Autodesk Fusion 360 part; units mm, degrees
(part 7 of 8)
  spline S2095 degree 3 poles (9.9865, -104.511) (10.0552, -104.4975) (10.0546, -104.4926) (9.9819, -104.494) knots 0 0 0 0 1 1 1 1
  spline S2096 degree 3 poles (9.9819, -104.494) (9.9092, -104.4954) (9.8779, -104.5067) (9.9001, -104.5241) knots 0 0 0 0 1 1 1 1
  spline S2097 degree 3 poles (10.4842, -104) (10.5266, -103.9973) (10.5607, -103.9881) (10.5588, -103.9733) knots 0 0 0 0 1 1 1 1
  spline S2098 degree 3 poles (10.5588, -103.9733) (10.557, -103.9584) (10.5998, -103.9381) (10.6487, -103.927) knots 0 0 0 0 1 1 1 1
  spline S2099 degree 3 poles (10.6487, -103.927) (10.7443, -103.9078) (10.7443, -103.9078) (10.6391, -103.9106) knots 0 0 0 0 1 1 1 1
  spline S2100 degree 3 poles (10.6391, -103.9106) (10.5819, -103.9151) (10.5379, -103.9256) (10.5397, -103.9404) knots 0 0 0 0 1 1 1 1
  spline S2101 degree 3 poles (10.5397, -103.9404) (10.5415, -103.9553) (10.5109, -103.9716) (10.4719, -103.9814) knots 0 0 0 0 1 1 1 1
  spline S2102 degree 3 poles (10.4719, -103.9814) (10.4109, -103.9964) (10.4137, -103.9986) (10.4842, -104) knots 0 0 0 0 1 1 1 1
  spline S2103 degree 3 poles (11.4822, -102.6711) (11.4877, -102.6755) (11.5273, -102.6706) (11.5685, -102.658) knots 0 0 0 0 1 1 1 1
  spline S2104 degree 3 poles (11.5685, -102.658) (11.6372, -102.6445) (11.6366, -102.6396) (11.5639, -102.641) knots 0 0 0 0 1 1 1 1
  spline S2105 degree 3 poles (11.5639, -102.641) (11.4912, -102.6424) (11.4599, -102.6537) (11.4822, -102.6711) knots 0 0 0 0 1 1 1 1
  spline S2106 degree 3 poles (12.3845, -101.6078) (12.4368, -101.6039) (12.4836, -101.5956) (12.4879, -101.5901) knots 0 0 0 0 1 1 1 1
  spline S2107 degree 3 poles (12.4879, -101.5901) (12.4923, -101.5845) (12.4586, -101.5761) (12.4128, -101.5717) knots 0 0 0 0 1 1 1 1
  spline S2108 degree 3 poles (12.4128, -101.5717) (12.367, -101.5672) (12.3203, -101.5755) (12.3094, -101.5894) knots 0 0 0 0 1 1 1 1
  spline S2109 degree 3 poles (12.3094, -101.5894) (12.2985, -101.6033) (12.3322, -101.6117) (12.3845, -101.6078) knots 0 0 0 0 1 1 1 1
  spline S2110 degree 3 poles (8.4693, -106.5847) (8.4748, -106.5891) (8.5145, -106.5842) (8.5556, -106.5716) knots 0 0 0 0 1 1 1 1
  spline S2111 degree 3 poles (8.5556, -106.5716) (8.6243, -106.5582) (8.6237, -106.5532) (8.551, -106.5546) knots 0 0 0 0 1 1 1 1
  spline S2112 degree 3 poles (8.551, -106.5546) (8.4783, -106.556) (8.447, -106.5674) (8.4693, -106.5847) knots 0 0 0 0 1 1 1 1
  spline S2113 degree 3 poles (15.3364, -97.8927) (15.3503, -97.9035) (15.3667, -97.894) (15.3692, -97.8736) knots 0 0 0 0 1 1 1 1
  spline S2114 degree 3 poles (15.3692, -97.8736) (15.3739, -97.8504) (15.3687, -97.8284) (15.3603, -97.8219) knots 0 0 0 0 1 1 1 1
  spline S2115 degree 3 poles (15.3603, -97.8219) (15.3548, -97.8175) (15.3405, -97.8243) (15.3275, -97.841) knots 0 0 0 0 1 1 1 1
  spline S2116 degree 3 poles (15.3275, -97.841) (15.3166, -97.8549) (15.3197, -97.8797) (15.3364, -97.8927) knots 0 0 0 0 1 1 1 1
  spline S2117 degree 3 poles (11.7356, -102.6677) (11.7879, -102.6637) (11.8346, -102.6555) (11.8411, -102.6472) knots 0 0 0 0 1 1 1 1
  spline S2118 degree 3 poles (11.8411, -102.6472) (11.8476, -102.6388) (11.8096, -102.6359) (11.7573, -102.6399) knots 0 0 0 0 1 1 1 1
  spline S2119 degree 3 poles (11.7573, -102.6399) (11.705, -102.6438) (11.6583, -102.652) (11.6517, -102.6604) knots 0 0 0 0 1 1 1 1
  spline S2120 degree 3 poles (11.6517, -102.6604) (11.6452, -102.6687) (11.6833, -102.6716) (11.7356, -102.6677) knots 0 0 0 0 1 1 1 1
  spline S2121 degree 3 poles (10.6627, -104.0007) (10.6683, -104.0051) (10.7036, -104.0058) (10.7376, -103.9965) knots 0 0 0 0 1 1 1 1
  spline S2122 degree 3 poles (10.7376, -103.9965) (10.7865, -103.9855) (10.7974, -103.9716) (10.7826, -103.9332) knots 0 0 0 0 1 1 1 1
  spline S2123 degree 3 poles (10.7826, -103.9332) (10.7718, -103.9069) (10.7635, -103.9004) (10.7638, -103.923) knots 0 0 0 0 1 1 1 1
  spline S2124 degree 3 poles (10.7638, -103.923) (10.7662, -103.9428) (10.7417, -103.9684) (10.7076, -103.9776) knots 0 0 0 0 1 1 1 1
  spline S2125 degree 3 poles (10.7076, -103.9776) (10.6758, -103.984) (10.6544, -103.9942) (10.6627, -104.0007) knots 0 0 0 0 1 1 1 1
  spline S2126 degree 3 poles (11.3676, -103.2532) (11.3815, -103.264) (11.4063, -103.261) (11.4172, -103.2471) knots 0 0 0 0 1 1 1 1
  spline S2127 degree 3 poles (11.4172, -103.2471) (11.4302, -103.2304) (11.425, -103.2084) (11.4111, -103.1976) knots 0 0 0 0 1 1 1 1
  spline S2128 degree 3 poles (11.4111, -103.1976) (11.3944, -103.1845) (11.3746, -103.187) (11.3616, -103.2037) knots 0 0 0 0 1 1 1 1
  spline S2129 degree 3 poles (11.3616, -103.2037) (11.3507, -103.2176) (11.351, -103.2401) (11.3676, -103.2532) knots 0 0 0 0 1 1 1 1
  spline S2130 degree 3 poles (12.6924, -101.5976) (12.741, -101.6042) (12.7806, -101.5994) (12.7788, -101.5845) knots 0 0 0 0 1 1 1 1
  spline S2131 degree 3 poles (12.7788, -101.5845) (12.7797, -101.5718) (12.7389, -101.5668) (12.6894, -101.5729) knots 0 0 0 0 1 1 1 1
  spline S2132 degree 3 poles (12.6894, -101.5729) (12.608, -101.5854) (12.6058, -101.5882) (12.6924, -101.5976) knots 0 0 0 0 1 1 1 1
  spline S2133 degree 3 poles (14.4902, -99.2909) (14.5124, -99.3083) (14.5344, -99.3031) (14.5369, -99.2827) knots 0 0 0 0 1 1 1 1
  spline S2134 degree 3 poles (14.5369, -99.2827) (14.5388, -99.2573) (14.5237, -99.2365) (14.5033, -99.234) knots 0 0 0 0 1 1 1 1
  spline S2135 degree 3 poles (14.5033, -99.234) (14.4448, -99.2286) (14.4401, -99.2518) (14.4902, -99.2909) knots 0 0 0 0 1 1 1 1
  spline S2136 degree 3 poles (10.9505, -103.8674) (10.956, -103.8717) (10.9956, -103.8668) (11.0368, -103.8542) knots 0 0 0 0 1 1 1 1
  spline S2137 degree 3 poles (11.0368, -103.8542) (11.1055, -103.8408) (11.1049, -103.8358) (11.0322, -103.8372) knots 0 0 0 0 1 1 1 1
  spline S2138 degree 3 poles (11.0322, -103.8372) (10.9595, -103.8386) (10.9282, -103.85) (10.9505, -103.8674) knots 0 0 0 0 1 1 1 1
  spline S2139 degree 3 poles (11.9636, -102.6623) (12.1053, -102.67) (12.929, -102.6644) (12.9983, -102.6559) knots 0 0 0 0 1 1 1 1
  spline S2140 degree 3 poles (12.9983, -102.6559) (13.1066, -102.6375) (13.0389, -102.6383) (12.4983, -102.6368) knots 0 0 0 0 1 1 1 1
  spline S2141 degree 3 poles (12.4983, -102.6368) (12.0911, -102.6366) (11.7888, -102.6511) (11.9636, -102.6623) knots 0 0 0 0 1 1 1 1
  spline S2142 degree 3 poles (8.921, -106.5795) (8.9266, -106.5839) (8.9662, -106.579) (9.0074, -106.5664) knots 0 0 0 0 1 1 1 1
  spline S2143 degree 3 poles (9.0074, -106.5664) (9.0761, -106.553) (9.0755, -106.548) (9.0028, -106.5494) knots 0 0 0 0 1 1 1 1
  spline S2144 degree 3 poles (9.0028, -106.5494) (8.9301, -106.5508) (8.8988, -106.5622) (8.921, -106.5795) knots 0 0 0 0 1 1 1 1
  spline S2145 degree 3 poles (10.9843, -103.9386) (10.9899, -103.9429) (11.0295, -103.9381) (11.0707, -103.9255) knots 0 0 0 0 1 1 1 1
  spline S2146 degree 3 poles (11.0707, -103.9255) (11.1394, -103.912) (11.1388, -103.9071) (11.0661, -103.9085) knots 0 0 0 0 1 1 1 1
  spline S2147 degree 3 poles (11.0661, -103.9085) (10.9934, -103.9098) (10.9621, -103.9212) (10.9843, -103.9386) knots 0 0 0 0 1 1 1 1
  spline S2148 degree 3 poles (11.5768, -103.2375) (11.5824, -103.2419) (11.622, -103.237) (11.6632, -103.2244) knots 0 0 0 0 1 1 1 1
  spline S2149 degree 3 poles (11.6632, -103.2244) (11.7319, -103.211) (11.7313, -103.206) (11.6586, -103.2074) knots 0 0 0 0 1 1 1 1
  spline S2150 degree 3 poles (11.6586, -103.2074) (11.5859, -103.2088) (11.5546, -103.2202) (11.5768, -103.2375) knots 0 0 0 0 1 1 1 1
  spline S2151 degree 3 poles (11.1371, -103.9952) (11.1541, -103.9906) (11.1869, -103.9715) (11.2071, -103.9515) knots 0 0 0 0 1 1 1 1
  spline S2152 degree 3 poles (11.2071, -103.9515) (11.2294, -103.9286) (11.2353, -103.9153) (11.2177, -103.915) knots 0 0 0 0 1 1 1 1
  spline S2153 degree 3 poles (11.2177, -103.915) (11.2007, -103.9196) (11.1678, -103.9387) (11.1477, -103.9588) knots 0 0 0 0 1 1 1 1
  spline S2154 degree 3 poles (11.1477, -103.9588) (11.1253, -103.9816) (11.1194, -103.9949) (11.1371, -103.9952) knots 0 0 0 0 1 1 1 1
  spline S2155 degree 3 poles (11.9296, -103.2445) (11.9351, -103.2488) (11.9747, -103.244) (12.0159, -103.2314) knots 0 0 0 0 1 1 1 1
  spline S2156 degree 3 poles (12.0159, -103.2314) (12.0846, -103.2179) (12.084, -103.213) (12.0113, -103.2144) knots 0 0 0 0 1 1 1 1
  spline S2157 degree 3 poles (12.0113, -103.2144) (11.9386, -103.2157) (11.9073, -103.2271) (11.9296, -103.2445) knots 0 0 0 0 1 1 1 1
  line L166 (17.1117, -96.7951) -> (17.1249, -96.9845)
  line L167 (17.1249, -96.9845) -> (17.1293, -96.7954)
  spline S2158 degree 3 poles (17.1293, -96.7954) (17.1324, -96.6367) (17.1245, -96.5723) (17.105, -96.5973) knots 0 0 0 0 1 1 1 1
  spline S2159 degree 3 poles (17.105, -96.5973) (17.1006, -96.6029) (17.1038, -96.6905) (17.1117, -96.7951) knots 0 0 0 0 1 1 1 1
  spline S2160 degree 3 poles (11.5786, -103.8656) (11.5841, -103.87) (11.6237, -103.8651) (11.6649, -103.8525) knots 0 0 0 0 1 1 1 1
  spline S2161 degree 3 poles (11.6649, -103.8525) (11.7336, -103.8391) (11.733, -103.8341) (11.6603, -103.8355) knots 0 0 0 0 1 1 1 1
  spline S2162 degree 3 poles (11.6603, -103.8355) (11.5876, -103.8369) (11.5563, -103.8483) (11.5786, -103.8656) knots 0 0 0 0 1 1 1 1
  spline S2163 degree 3 poles (13.3873, -101.6078) (13.3929, -101.6122) (13.4325, -101.6073) (13.4737, -101.5947) knots 0 0 0 0 1 1 1 1
  spline S2164 degree 3 poles (13.4737, -101.5947) (13.5424, -101.5812) (13.5418, -101.5763) (13.4691, -101.5777) knots 0 0 0 0 1 1 1 1
  spline S2165 degree 3 poles (13.4691, -101.5777) (13.3964, -101.5791) (13.3651, -101.5904) (13.3873, -101.6078) knots 0 0 0 0 1 1 1 1
  spline S2166 degree 3 poles (12.1554, -103.2419) (12.161, -103.2462) (12.2006, -103.2414) (12.2418, -103.2288) knots 0 0 0 0 1 1 1 1
  spline S2167 degree 3 poles (12.2418, -103.2288) (12.3105, -103.2153) (12.3099, -103.2104) (12.2372, -103.2118) knots 0 0 0 0 1 1 1 1
  spline S2168 degree 3 poles (12.2372, -103.2118) (12.1645, -103.2131) (12.1332, -103.2245) (12.1554, -103.2419) knots 0 0 0 0 1 1 1 1
  spline S2169 degree 3 poles (7.6066, -109.1788) (7.6121, -109.1831) (7.6517, -109.1783) (7.6929, -109.1657) knots 0 0 0 0 1 1 1 1
  spline S2170 degree 3 poles (7.6929, -109.1657) (7.7616, -109.1522) (7.761, -109.1473) (7.6883, -109.1486) knots 0 0 0 0 1 1 1 1
  spline S2171 degree 3 poles (7.6883, -109.1486) (7.6156, -109.15) (7.5843, -109.1614) (7.6066, -109.1788) knots 0 0 0 0 1 1 1 1
  spline S2172 degree 3 poles (11.832, -103.8622) (11.8843, -103.8583) (11.931, -103.85) (11.9375, -103.8417) knots 0 0 0 0 1 1 1 1
  spline S2173 degree 3 poles (11.9375, -103.8417) (11.944, -103.8333) (11.906, -103.8305) (11.8537, -103.8344) knots 0 0 0 0 1 1 1 1
  spline S2174 degree 3 poles (11.8537, -103.8344) (11.8014, -103.8383) (11.7547, -103.8465) (11.7481, -103.8549) knots 0 0 0 0 1 1 1 1
  spline S2175 degree 3 poles (11.7481, -103.8549) (11.7416, -103.8632) (11.7797, -103.8661) (11.832, -103.8622) knots 0 0 0 0 1 1 1 1
  line L168 (17.1131, -97.1141) -> (17.1358, -97.2168)
  line L169 (17.1358, -97.2168) -> (17.1329, -97.1116)
  spline S2176 degree 3 poles (17.1329, -97.1116) (17.1284, -97.0544) (17.1223, -97.0049) (17.1168, -97.0005) knots 0 0 0 0 1 1 1 1
  spline S2177 degree 3 poles (17.1168, -97.0005) (17.0945, -96.9832) (17.0938, -97.0184) (17.1131, -97.1141) knots 0 0 0 0 1 1 1 1
  spline S2178 degree 3 poles (13.3509, -101.9868) (13.4258, -101.9826) (13.4983, -101.9586) (13.5129, -101.9342) knots 0 0 0 0 1 1 1 1
  spline S2179 degree 3 poles (13.5129, -101.9342) (13.5433, -101.8953) (13.5405, -101.8931) (13.4984, -101.9184) knots 0 0 0 0 1 1 1 1
  spline S2180 degree 3 poles (13.4984, -101.9184) (13.4726, -101.9341) (13.4002, -101.9581) (13.3364, -101.971) knots 0 0 0 0 1 1 1 1
  line L170 (13.3364, -101.971) -> (13.2237, -101.9948)
  line L171 (13.2237, -101.9948) -> (13.3509, -101.9868)
  spline S2181 degree 3 poles (13.6968, -101.5899) (13.7528, -101.5755) (13.8057, -101.5766) (13.8196, -101.5874) knots 0 0 0 0 1 1 1 1
  spline S2182 degree 3 poles (13.8196, -101.5874) (13.8286, -101.5989) (13.8512, -101.5986) (13.8697, -101.5863) knots 0 0 0 0 1 1 1 1
  spline S2183 degree 3 poles (13.8697, -101.5863) (13.8883, -101.574) (13.8964, -101.5579) (13.8881, -101.5514) knots 0 0 0 0 1 1 1 1
  spline S2184 degree 3 poles (13.8881, -101.5514) (13.8631, -101.5318) (13.6303, -101.5604) (13.6108, -101.5854) knots 0 0 0 0 1 1 1 1
  spline S2185 degree 3 poles (13.6108, -101.5854) (13.6027, -101.6015) (13.638, -101.6022) (13.6968, -101.5899) knots 0 0 0 0 1 1 1 1
  spline S2186 degree 3 poles (12.3813, -103.2393) (12.3869, -103.2436) (12.4265, -103.2388) (12.4676, -103.2262) knots 0 0 0 0 1 1 1 1
  spline S2187 degree 3 poles (12.4676, -103.2262) (12.5364, -103.2127) (12.5358, -103.2078) (12.463, -103.2092) knots 0 0 0 0 1 1 1 1
  spline S2188 degree 3 poles (12.463, -103.2092) (12.3903, -103.2105) (12.3591, -103.2219) (12.3813, -103.2393) knots 0 0 0 0 1 1 1 1
  spline S2189 degree 3 poles (7.7829, -109.1823) (7.7885, -109.1866) (7.8281, -109.1817) (7.8693, -109.1691) knots 0 0 0 0 1 1 1 1
  spline S2190 degree 3 poles (7.8693, -109.1691) (7.938, -109.1557) (7.9374, -109.1507) (7.8647, -109.1521) knots 0 0 0 0 1 1 1 1
  spline S2191 degree 3 poles (7.8647, -109.1521) (7.7919, -109.1535) (7.7607, -109.1649) (7.7829, -109.1823) knots 0 0 0 0 1 1 1 1
  spline S2192 degree 3 poles (17.1127, -97.3152) (17.1289, -97.3861) (17.1339, -97.3855) (17.1325, -97.3128) knots 0 0 0 0 1 1 1 1
  spline S2193 degree 3 poles (17.1325, -97.3128) (17.1326, -97.2725) (17.1277, -97.2329) (17.1222, -97.2286) knots 0 0 0 0 1 1 1 1
  spline S2194 degree 3 poles (17.1222, -97.2286) (17.0999, -97.2112) (17.0964, -97.2443) (17.1127, -97.3152) knots 0 0 0 0 1 1 1 1
  spline S2195 degree 3 poles (11.9808, -103.8665) (11.9864, -103.8709) (12.026, -103.866) (12.0671, -103.8534) knots 0 0 0 0 1 1 1 1
  spline S2196 degree 3 poles (12.0671, -103.8534) (12.1359, -103.8399) (12.1353, -103.835) (12.0625, -103.8364) knots 0 0 0 0 1 1 1 1
  spline S2197 degree 3 poles (12.0625, -103.8364) (11.9898, -103.8378) (11.9586, -103.8491) (11.9808, -103.8665) knots 0 0 0 0 1 1 1 1
  spline S2198 degree 3 poles (12.5577, -103.2428) (12.5632, -103.2471) (12.6028, -103.2423) (12.644, -103.2297) knots 0 0 0 0 1 1 1 1
  spline S2199 degree 3 poles (12.644, -103.2297) (12.7127, -103.2162) (12.7121, -103.2112) (12.6394, -103.2126) knots 0 0 0 0 1 1 1 1
  spline S2200 degree 3 poles (12.6394, -103.2126) (12.5667, -103.214) (12.5354, -103.2254) (12.5577, -103.2428) knots 0 0 0 0 1 1 1 1
  line L172 (17.1122, -97.5163) -> (17.1349, -97.6191)
  line L173 (17.1349, -97.6191) -> (17.1321, -97.5139)
  spline S2201 degree 3 poles (17.1321, -97.5139) (17.1275, -97.4566) (17.1215, -97.4071) (17.1159, -97.4028) knots 0 0 0 0 1 1 1 1
  spline S2202 degree 3 poles (17.1159, -97.4028) (17.0937, -97.3854) (17.093, -97.4207) (17.1122, -97.5163) knots 0 0 0 0 1 1 1 1
  spline S2203 degree 3 poles (8.0088, -109.1797) (8.0143, -109.184) (8.054, -109.1791) (8.0951, -109.1665) knots 0 0 0 0 1 1 1 1
  spline S2204 degree 3 poles (8.0951, -109.1665) (8.1639, -109.1531) (8.1632, -109.1481) (8.0905, -109.1495) knots 0 0 0 0 1 1 1 1
  spline S2205 degree 3 poles (8.0905, -109.1495) (8.0178, -109.1509) (7.9865, -109.1623) (8.0088, -109.1797) knots 0 0 0 0 1 1 1 1
  spline S2206 degree 3 poles (13.4227, -102.2846) (13.4431, -102.2871) (13.4679, -102.2841) (13.4744, -102.2757) knots 0 0 0 0 1 1 1 1
  spline S2207 degree 3 poles (13.4744, -102.2757) (13.4787, -102.2702) (13.4692, -102.2537) (13.4553, -102.2429) knots 0 0 0 0 1 1 1 1
  spline S2208 degree 3 poles (13.4553, -102.2429) (13.4386, -102.2298) (13.4166, -102.2351) (13.4036, -102.2517) knots 0 0 0 0 1 1 1 1
  spline S2209 degree 3 poles (13.4036, -102.2517) (13.3927, -102.2656) (13.3995, -102.2799) (13.4227, -102.2846) knots 0 0 0 0 1 1 1 1
  spline S2210 degree 3 poles (13.8512, -101.7017) (13.8568, -101.706) (13.8964, -101.7011) (13.9376, -101.6885) knots 0 0 0 0 1 1 1 1
  spline S2211 degree 3 poles (13.9376, -101.6885) (14.0063, -101.6751) (14.0057, -101.6701) (13.933, -101.6715) knots 0 0 0 0 1 1 1 1
  spline S2212 degree 3 poles (13.933, -101.6715) (13.8603, -101.6729) (13.829, -101.6843) (13.8512, -101.7017) knots 0 0 0 0 1 1 1 1
  spline S2213 degree 3 poles (12.2067, -103.8639) (12.2122, -103.8683) (12.2518, -103.8634) (12.293, -103.8508) knots 0 0 0 0 1 1 1 1
  spline S2214 degree 3 poles (12.293, -103.8508) (12.3617, -103.8373) (12.3611, -103.8324) (12.2884, -103.8338) knots 0 0 0 0 1 1 1 1
  spline S2215 degree 3 poles (12.2884, -103.8338) (12.2157, -103.8352) (12.1844, -103.8465) (12.2067, -103.8639) knots 0 0 0 0 1 1 1 1
  spline S2216 degree 3 poles (14.0919, -101.5942) (14.1414, -101.5881) (14.1848, -101.5727) (14.1835, -101.5628) knots 0 0 0 0 1 1 1 1
  spline S2217 degree 3 poles (14.1835, -101.5628) (14.1799, -101.5331) (14.0456, -101.5446) (14.0195, -101.578) knots 0 0 0 0 1 1 1 1
  spline S2218 degree 3 poles (14.0195, -101.578) (14.0065, -101.5946) (14.0374, -101.6009) (14.0919, -101.5942) knots 0 0 0 0 1 1 1 1
  spline S2219 degree 3 poles (17.1118, -97.7174) (17.1281, -97.7883) (17.133, -97.7877) (17.1316, -97.715) knots 0 0 0 0 1 1 1 1
  spline S2220 degree 3 poles (17.1316, -97.715) (17.1317, -97.6748) (17.1268, -97.6351) (17.1213, -97.6308) knots 0 0 0 0 1 1 1 1
  spline S2221 degree 3 poles (17.1213, -97.6308) (17.099, -97.6134) (17.0956, -97.6465) (17.1118, -97.7174) knots 0 0 0 0 1 1 1 1
  spline S2222 degree 3 poles (12.7835, -103.2402) (12.7891, -103.2445) (12.8287, -103.2397) (12.8699, -103.2271) knots 0 0 0 0 1 1 1 1
  spline S2223 degree 3 poles (12.8699, -103.2271) (12.9386, -103.2136) (12.938, -103.2086) (12.8653, -103.21) knots 0 0 0 0 1 1 1 1
  spline S2224 degree 3 poles (12.8653, -103.21) (12.7926, -103.2114) (12.7613, -103.2228) (12.7835, -103.2402) knots 0 0 0 0 1 1 1 1
  spline S2225 degree 3 poles (17.0444, -97.8438) (17.0917, -97.8405) (17.104, -97.8993) (17.1048, -98.1103) knots 0 0 0 0 1 1 1 1
  spline S2226 degree 3 poles (17.1048, -98.1103) (17.1054, -98.2586) (17.1134, -98.3857) (17.1218, -98.3923) knots 0 0 0 0 1 1 1 1
  spline S2227 degree 3 poles (17.1218, -98.3923) (17.1357, -98.4031) (17.1399, -98.1513) (17.1287, -97.8963) knots 0 0 0 0 1 1 1 1
  spline S2228 degree 3 poles (17.1287, -97.8963) (17.1267, -97.8186) (17.0424, -97.7661) (17.0033, -97.8162) knots 0 0 0 0 1 1 1 1
  spline S2229 degree 3 poles (17.0033, -97.8162) (16.9881, -97.8356) (17.0042, -97.8437) (17.0444, -97.8438) knots 0 0 0 0 1 1 1 1
  spline S2230 degree 3 poles (8.2347, -109.1771) (8.2402, -109.1814) (8.2798, -109.1765) (8.321, -109.1639) knots 0 0 0 0 1 1 1 1
  spline S2231 degree 3 poles (8.321, -109.1639) (8.3897, -109.1505) (8.3891, -109.1455) (8.3164, -109.1469) knots 0 0 0 0 1 1 1 1
  spline S2232 degree 3 poles (8.3164, -109.1469) (8.2437, -109.1483) (8.2124, -109.1597) (8.2347, -109.1771) knots 0 0 0 0 1 1 1 1
  spline S2233 degree 3 poles (12.4601, -103.8604) (12.5124, -103.8565) (12.5591, -103.8483) (12.5656, -103.8399) knots 0 0 0 0 1 1 1 1
  spline S2234 degree 3 poles (12.5656, -103.8399) (12.5721, -103.8316) (12.5341, -103.8287) (12.4818, -103.8327) knots 0 0 0 0 1 1 1 1
  spline S2235 degree 3 poles (12.4818, -103.8327) (12.4295, -103.8366) (12.3828, -103.8448) (12.3762, -103.8532) knots 0 0 0 0 1 1 1 1
  spline S2236 degree 3 poles (12.3762, -103.8532) (12.3697, -103.8615) (12.4078, -103.8644) (12.4601, -103.8604) knots 0 0 0 0 1 1 1 1
  spline S2237 degree 3 poles (14.3119, -101.6049) (14.3576, -101.6093) (14.4022, -101.6038) (14.4109, -101.5927) knots 0 0 0 0 1 1 1 1
  spline S2238 degree 3 poles (14.4109, -101.5927) (14.4217, -101.5788) (14.3924, -101.5648) (14.3466, -101.5604) knots 0 0 0 0 1 1 1 1
  spline S2239 degree 3 poles (14.3466, -101.5604) (14.3008, -101.556) (14.2563, -101.5614) (14.2476, -101.5726) knots 0 0 0 0 1 1 1 1
  spline S2240 degree 3 poles (14.2476, -101.5726) (14.2367, -101.5865) (14.2661, -101.6005) (14.3119, -101.6049) knots 0 0 0 0 1 1 1 1
  spline S2241 degree 3 poles (14.2535, -101.7025) (14.259, -101.7069) (14.2986, -101.702) (14.3398, -101.6894) knots 0 0 0 0 1 1 1 1
  spline S2242 degree 3 poles (14.3398, -101.6894) (14.4085, -101.676) (14.4079, -101.671) (14.3352, -101.6724) knots 0 0 0 0 1 1 1 1
  spline S2243 degree 3 poles (14.3352, -101.6724) (14.2625, -101.6738) (14.2312, -101.6852) (14.2535, -101.7025) knots 0 0 0 0 1 1 1 1
  spline S2244 degree 3 poles (12.6089, -103.8648) (12.6145, -103.8691) (12.6541, -103.8643) (12.6952, -103.8517) knots 0 0 0 0 1 1 1 1
  spline S2245 degree 3 poles (12.6952, -103.8517) (12.764, -103.8382) (12.7634, -103.8333) (12.6906, -103.8347) knots 0 0 0 0 1 1 1 1
  spline S2246 degree 3 poles (12.6906, -103.8347) (12.6179, -103.836) (12.5867, -103.8474) (12.6089, -103.8648) knots 0 0 0 0 1 1 1 1
  spline S2247 degree 3 poles (12.7852, -103.8683) (12.7908, -103.8726) (12.8304, -103.8678) (12.8716, -103.8552) knots 0 0 0 0 1 1 1 1
  spline S2248 degree 3 poles (12.8716, -103.8552) (12.9403, -103.8417) (12.9397, -103.8367) (12.867, -103.8381) knots 0 0 0 0 1 1 1 1
  spline S2249 degree 3 poles (12.867, -103.8381) (12.7943, -103.8395) (12.763, -103.8509) (12.7852, -103.8683) knots 0 0 0 0 1 1 1 1
  spline S2250 degree 3 poles (14.5641, -101.6945) (14.6248, -101.6972) (14.6765, -101.6883) (14.6752, -101.6784) knots 0 0 0 0 1 1 1 1
  spline S2251 degree 3 poles (14.6752, -101.6784) (14.6734, -101.6635) (14.6205, -101.6625) (14.5611, -101.6698) knots 0 0 0 0 1 1 1 1
  line L174 (14.5611, -101.6698) -> (14.4478, -101.6887)
  line L175 (14.4478, -101.6887) -> (14.5641, -101.6945)
  spline S2252 degree 3 poles (14.5801, -101.5996) (14.5968, -101.6126) (14.6222, -101.6145) (14.6392, -101.6099) knots 0 0 0 0 1 1 1 1
  spline S2253 degree 3 poles (14.6392, -101.6099) (14.6584, -101.6025) (14.656, -101.5827) (14.6337, -101.5654) knots 0 0 0 0 1 1 1 1
  spline S2254 degree 3 poles (14.6337, -101.5654) (14.6115, -101.548) (14.5833, -101.5439) (14.5725, -101.5578) knots 0 0 0 0 1 1 1 1
  spline S2255 degree 3 poles (14.5725, -101.5578) (14.5638, -101.5689) (14.5662, -101.5887) (14.5801, -101.5996) knots 0 0 0 0 1 1 1 1
  spline S2256 degree 3 poles (17.1029, -98.6685) (17.1102, -99.0144) (17.1314, -99.0847) (17.1327, -98.7679) knots 0 0 0 0 1 1 1 1
  spline S2257 degree 3 poles (17.1327, -98.7679) (17.1326, -98.5216) (17.123, -98.4022) (17.1041, -98.4321) knots 0 0 0 0 1 1 1 1
  spline S2258 degree 3 poles (17.1041, -98.4321) (17.1025, -98.4399) (17.1026, -98.5429) (17.1029, -98.6685) knots 0 0 0 0 1 1 1 1
  spline S2259 degree 3 poles (14.7634, -101.5369) (14.7708, -101.5561) (14.8095, -101.5639) (14.8506, -101.5513) knots 0 0 0 0 1 1 1 1
  spline S2260 degree 3 poles (14.8506, -101.5513) (14.9166, -101.5357) (14.9188, -101.5329) (14.8559, -101.5331) knots 0 0 0 0 1 1 1 1
  spline S2261 degree 3 poles (14.8559, -101.5331) (14.8157, -101.533) (14.7814, -101.5196) (14.7818, -101.502) knots 0 0 0 0 1 1 1 1
  spline S2262 degree 3 poles (14.7818, -101.502) (14.7772, -101.4849) (14.771, -101.4756) (14.7623, -101.4867) knots 0 0 0 0 1 1 1 1
  spline S2263 degree 3 poles (14.7623, -101.4867) (14.7558, -101.4951) (14.756, -101.5177) (14.7634, -101.5369) knots 0 0 0 0 1 1 1 1
  spline S2264 degree 3 poles (14.3143, -102.1977) (14.3198, -102.2021) (14.3594, -102.1972) (14.4006, -102.1846) knots 0 0 0 0 1 1 1 1
  spline S2265 degree 3 poles (14.4006, -102.1846) (14.4693, -102.1711) (14.4687, -102.1662) (14.396, -102.1676) knots 0 0 0 0 1 1 1 1
  spline S2266 degree 3 poles (14.396, -102.1676) (14.3233, -102.169) (14.292, -102.1803) (14.3143, -102.1977) knots 0 0 0 0 1 1 1 1
  spline S2267 degree 3 poles (14.9337, -101.4908) (14.9411, -101.51) (14.9748, -101.5185) (15.0067, -101.512) knots 0 0 0 0 1 1 1 1
  spline S2268 degree 3 poles (15.0067, -101.512) (15.0534, -101.5038) (15.0664, -101.4871) (15.0551, -101.4558) knots 0 0 0 0 1 1 1 1
  spline S2269 degree 3 poles (15.0551, -101.4558) (15.0471, -101.4317) (15.0322, -101.4335) (15.0176, -101.4579) knots 0 0 0 0 1 1 1 1
  spline S2270 degree 3 poles (15.0176, -101.4579) (15.008, -101.4817) (14.9832, -101.4848) (14.9681, -101.464) knots 0 0 0 0 1 1 1 1
  spline S2271 degree 3 poles (14.9681, -101.464) (14.9335, -101.428) (14.9149, -101.4404) (14.9337, -101.4908) knots 0 0 0 0 1 1 1 1
  spline S2272 degree 3 poles (17.0258, -98.8589) (17.042, -98.9298) (17.047, -98.9292) (17.0456, -98.8565) knots 0 0 0 0 1 1 1 1
  spline S2273 degree 3 poles (17.0456, -98.8565) (17.0457, -98.8163) (17.0408, -98.7767) (17.0352, -98.7723) knots 0 0 0 0 1 1 1 1
  spline S2274 degree 3 poles (17.0352, -98.7723) (17.013, -98.755) (17.0095, -98.7881) (17.0258, -98.8589) knots 0 0 0 0 1 1 1 1
  line L176 (16.2989, -99.8982) -> (16.2863, -100.0003)
  line L177 (16.2863, -100.0003) -> (16.3211, -99.9156)
  spline S2275 degree 3 poles (16.3211, -99.9156) (16.3625, -99.8225) (16.3638, -99.7922) (16.3341, -99.7959) knots 0 0 0 0 1 1 1 1
  spline S2276 degree 3 poles (16.3341, -99.7959) (16.3242, -99.7971) (16.307, -99.8419) (16.2989, -99.8982) knots 0 0 0 0 1 1 1 1
  spline S2277 degree 3 poles (15.104, -101.4448) (15.1114, -101.464) (15.15, -101.4718) (15.1912, -101.4592) knots 0 0 0 0 1 1 1 1
  spline S2278 degree 3 poles (15.1912, -101.4592) (15.2571, -101.4436) (15.2593, -101.4408) (15.1965, -101.441) knots 0 0 0 0 1 1 1 1
  spline S2279 degree 3 poles (15.1965, -101.441) (15.1563, -101.4409) (15.122, -101.4275) (15.1223, -101.4099) knots 0 0 0 0 1 1 1 1
  spline S2280 degree 3 poles (15.1223, -101.4099) (15.1177, -101.3928) (15.1115, -101.3836) (15.1028, -101.3947) knots 0 0 0 0 1 1 1 1
  spline S2281 degree 3 poles (15.1028, -101.3947) (15.0963, -101.403) (15.0966, -101.4256) (15.104, -101.4448) knots 0 0 0 0 1 1 1 1
  spline S2282 degree 3 poles (11.2181, -106.579) (11.3251, -106.591) (11.353, -106.5725) (11.3219, -106.5034) knots 0 0 0 0 1 1 1 1
  spline S2283 degree 3 poles (11.3219, -106.5034) (11.3139, -106.4792) (11.3034, -106.4755) (11.3086, -106.4975) knots 0 0 0 0 1 1 1 1
  spline S2284 degree 3 poles (11.3086, -106.4975) (11.3088, -106.5201) (11.2689, -106.5426) (11.22, -106.5536) knots 0 0 0 0 1 1 1 1
  spline S2285 degree 3 poles (11.22, -106.5536) (11.1287, -106.5673) (11.1315, -106.5695) (11.2181, -106.579) knots 0 0 0 0 1 1 1 1
  spline S2286 degree 3 poles (15.2779, -101.4285) (15.2835, -101.4328) (15.3132, -101.4292) (15.3451, -101.4227) knots 0 0 0 0 1 1 1 1
  spline S2287 degree 3 poles (15.3451, -101.4227) (15.389, -101.4123) (15.3949, -101.399) (15.3699, -101.3795) knots 0 0 0 0 1 1 1 1
  spline S2288 degree 3 poles (15.3699, -101.3795) (15.3477, -101.3621) (15.3179, -101.3657) (15.3006, -101.388) knots 0 0 0 0 1 1 1 1
  spline S2289 degree 3 poles (15.3006, -101.388) (15.2854, -101.4074) (15.2751, -101.4263) (15.2779, -101.4285) knots 0 0 0 0 1 1 1 1
  line L178 (17.1148, -99.1747) -> (17.1375, -99.2775)
  line L179 (17.1375, -99.2775) -> (17.1346, -99.1723)
  spline S2290 degree 3 poles (17.1346, -99.1723) (17.1301, -99.115) (17.124, -99.0655) (17.1185, -99.0612) knots 0 0 0 0 1 1 1 1
  spline S2291 degree 3 poles (17.1185, -99.0612) (17.0962, -99.0438) (17.0955, -99.0791) (17.1148, -99.1747) knots 0 0 0 0 1 1 1 1
  spline S2292 degree 3 poles (14.7877, -102.1647) (14.7933, -102.1691) (14.8329, -102.1642) (14.8741, -102.1516) knots 0 0 0 0 1 1 1 1
  spline S2293 degree 3 poles (14.8741, -102.1516) (14.9428, -102.1381) (14.9422, -102.1332) (14.8695, -102.1346) knots 0 0 0 0 1 1 1 1
  spline S2294 degree 3 poles (14.8695, -102.1346) (14.7968, -102.136) (14.7655, -102.1473) (14.7877, -102.1647) knots 0 0 0 0 1 1 1 1
  spline S2295 degree 3 poles (10.4188, -107.8885) (10.435, -107.9594) (10.44, -107.9588) (10.4386, -107.8861) knots 0 0 0 0 1 1 1 1
  spline S2296 degree 3 poles (10.4386, -107.8861) (10.4372, -107.8134) (10.4258, -107.7821) (10.4085, -107.8043) knots 0 0 0 0 1 1 1 1
  spline S2297 degree 3 poles (10.4085, -107.8043) (10.4041, -107.8099) (10.409, -107.8495) (10.4188, -107.8885) knots 0 0 0 0 1 1 1 1
  spline S2298 degree 3 poles (15.408, -101.4854) (15.4136, -101.4897) (15.4532, -101.4849) (15.4944, -101.4723) knots 0 0 0 0 1 1 1 1
  spline S2299 degree 3 poles (15.4944, -101.4723) (15.5631, -101.4588) (15.5625, -101.4538) (15.4898, -101.4552) knots 0 0 0 0 1 1 1 1
  spline S2300 degree 3 poles (15.4898, -101.4552) (15.4171, -101.4566) (15.3858, -101.468) (15.408, -101.4854) knots 0 0 0 0 1 1 1 1
  spline S2301 degree 3 poles (17.105, -99.5655) (17.1084, -99.7159) (17.1052, -99.8746) (17.098, -99.9182) knots 0 0 0 0 1 1 1 1
  spline S2302 degree 3 poles (17.098, -99.9182) (17.0908, -99.9618) (17.0988, -99.986) (17.1118, -99.9693) knots 0 0 0 0 1 1 1 1
  spline S2303 degree 3 poles (17.1118, -99.9693) (17.1336, -99.9415) (17.1436, -99.4703) (17.1269, -99.314) knots 0 0 0 0 1 1 1 1
  spline S2304 degree 3 poles (17.1269, -99.314) (17.1117, -99.1902) (17.1006, -99.3248) (17.105, -99.5655) knots 0 0 0 0 1 1 1 1
  spline S2305 degree 3 poles (15.6117, -101.4654) (15.6339, -101.4828) (15.6559, -101.4776) (15.6584, -101.4571) knots 0 0 0 0 1 1 1 1
  spline S2306 degree 3 poles (15.6584, -101.4571) (15.6631, -101.4339) (15.6523, -101.4076) (15.6356, -101.3946) knots 0 0 0 0 1 1 1 1
  spline S2307 degree 3 poles (15.6356, -101.3946) (15.6217, -101.3837) (15.6019, -101.3862) (15.5889, -101.4028) knots 0 0 0 0 1 1 1 1
  spline S2308 degree 3 poles (15.5889, -101.4028) (15.578, -101.4167) (15.5866, -101.4458) (15.6117, -101.4654) knots 0 0 0 0 1 1 1 1
  spline S2309 degree 3 poles (15.2986, -102.0266) (15.3041, -102.0309) (15.3437, -102.0261) (15.3849, -102.0135) knots 0 0 0 0 1 1 1 1
  spline S2310 degree 3 poles (15.3849, -102.0135) (15.4536, -102) (15.453, -101.9951) (15.3803, -101.9965) knots 0 0 0 0 1 1 1 1
  spline S2311 degree 3 poles (15.3803, -101.9965) (15.3076, -101.9978) (15.2763, -102.0092) (15.2986, -102.0266) knots 0 0 0 0 1 1 1 1
  spline S2312 degree 3 poles (16.2978, -100.8106) (16.3287, -100.8169) (16.3569, -100.821) (16.3612, -100.8154) knots 0 0 0 0 1 1 1 1
  spline S2313 degree 3 poles (16.3612, -100.8154) (16.3656, -100.8099) (16.3505, -100.7891) (16.3282, -100.7717) knots 0 0 0 0 1 1 1 1
  spline S2314 degree 3 poles (16.3282, -100.7717) (16.306, -100.7543) (16.2778, -100.7503) (16.2648, -100.7669) knots 0 0 0 0 1 1 1 1
  spline S2315 degree 3 poles (16.2648, -100.7669) (16.2539, -100.7808) (16.2691, -100.8016) (16.2978, -100.8106) knots 0 0 0 0 1 1 1 1
  spline S2316 degree 3 poles (17.0319, -100.1575) (17.0237, -100.2138) (17.0274, -100.2435) (17.0383, -100.2296) knots 0 0 0 0 1 1 1 1
  spline S2317 degree 3 poles (17.0383, -100.2296) (17.0513, -100.213) (17.0672, -100.1582) (17.0754, -100.1019) knots 0 0 0 0 1 1 1 1
  spline S2318 degree 3 poles (17.0754, -100.1019) (17.0835, -100.0456) (17.082, -100.0132) (17.069, -100.0298) knots 0 0 0 0 1 1 1 1
  spline S2319 degree 3 poles (17.069, -100.0298) (17.0582, -100.0437) (17.0401, -100.1012) (17.0319, -100.1575) knots 0 0 0 0 1 1 1 1
  spline S2320 degree 3 poles (15.6391, -101.9345) (15.6447, -101.9389) (15.6843, -101.934) (15.7255, -101.9214) knots 0 0 0 0 1 1 1 1
  spline S2321 degree 3 poles (15.7255, -101.9214) (15.7942, -101.9079) (15.7936, -101.903) (15.7209, -101.9044) knots 0 0 0 0 1 1 1 1
  spline S2322 degree 3 poles (15.7209, -101.9044) (15.6481, -101.9058) (15.6169, -101.9171) (15.6391, -101.9345) knots 0 0 0 0 1 1 1 1
  spline S2323 degree 3 poles (16.9711, -100.3786) (16.9676, -100.4117) (16.9772, -100.4281) (16.988, -100.4142) knots 0 0 0 0 1 1 1 1
  spline S2324 degree 3 poles (16.988, -100.4142) (17.0011, -100.3976) (17.0111, -100.3561) (17.0145, -100.323) knots 0 0 0 0 1 1 1 1
  spline S2325 degree 3 poles (17.0145, -100.323) (17.018, -100.2899) (17.0106, -100.2707) (16.9976, -100.2874) knots 0 0 0 0 1 1 1 1
  spline S2326 degree 3 poles (16.9976, -100.2874) (16.9867, -100.3013) (16.9746, -100.3455) (16.9711, -100.3786) knots 0 0 0 0 1 1 1 1
  spline S2327 degree 3 poles (16.9025, -100.6384) (16.899, -100.6715) (16.9085, -100.6879) (16.9194, -100.674) knots 0 0 0 0 1 1 1 1
  spline S2328 degree 3 poles (16.9194, -100.674) (16.9324, -100.6573) (16.9424, -100.6159) (16.9459, -100.5828) knots 0 0 0 0 1 1 1 1
  spline S2329 degree 3 poles (16.9459, -100.5828) (16.9494, -100.5497) (16.942, -100.5305) (16.929, -100.5472) knots 0 0 0 0 1 1 1 1
  spline S2330 degree 3 poles (16.929, -100.5472) (16.9181, -100.5611) (16.9059, -100.6053) (16.9025, -100.6384) knots 0 0 0 0 1 1 1 1
  spline S2331 degree 3 poles (8.0158, -112.1846) (8.0864, -112.186) (8.1514, -112.1831) (8.1557, -112.1775) knots 0 0 0 0 1 1 1 1
  spline S2332 degree 3 poles (8.1557, -112.1775) (8.1622, -112.1692) (8.1081, -112.1582) (8.0376, -112.1568) knots 0 0 0 0 1 1 1 1
  spline S2333 degree 3 poles (8.0376, -112.1568) (7.9642, -112.1533) (7.902, -112.1584) (7.8977, -112.164) knots 0 0 0 0 1 1 1 1
  spline S2334 degree 3 poles (7.8977, -112.164) (7.8912, -112.1723) (7.9425, -112.1811) (8.0158, -112.1846) knots 0 0 0 0 1 1 1 1
  spline S2335 degree 3 poles (16.0115, -101.8762) (16.035, -101.8633) (16.0518, -101.8361) (16.0499, -101.8212) knots 0 0 0 0 1 1 1 1
  spline S2336 degree 3 poles (16.0499, -101.8212) (16.0503, -101.8036) (16.0289, -101.8138) (16.0078, -101.8465) knots 0 0 0 0 1 1 1 1
  spline S2337 degree 3 poles (16.0078, -101.8465) (15.9839, -101.8771) (15.9857, -101.892) (16.0115, -101.8762) knots 0 0 0 0 1 1 1 1
  spline S2338 degree 3 poles (16.8416, -100.8595) (16.8335, -100.9158) (16.8371, -100.9455) (16.848, -100.9316) knots 0 0 0 0 1 1 1 1
  spline S2339 degree 3 poles (16.848, -100.9316) (16.861, -100.9149) (16.8769, -100.8602) (16.8851, -100.8039) knots 0 0 0 0 1 1 1 1
  spline S2340 degree 3 poles (16.8851, -100.8039) (16.8933, -100.7476) (16.8918, -100.7151) (16.8787, -100.7318) knots 0 0 0 0 1 1 1 1
  spline S2341 degree 3 poles (16.8787, -100.7318) (16.8679, -100.7457) (16.8498, -100.8032) (16.8416, -100.8595) knots 0 0 0 0 1 1 1 1
  spline S2342 degree 3 poles (16.1804, -101.7173) (16.2055, -101.6966) (16.2403, -101.6521) (16.2564, -101.62) knots 0 0 0 0 1 1 1 1
  spline S2343 degree 3 poles (16.2564, -101.62) (16.2677, -101.5884) (16.2447, -101.6063) (16.2035, -101.6591) knots 0 0 0 0 1 1 1 1
  spline S2344 degree 3 poles (16.2035, -101.6591) (16.1622, -101.712) (16.1504, -101.7385) (16.1804, -101.7173) knots 0 0 0 0 1 1 1 1
  spline S2345 degree 3 poles (16.74, -101.0755) (16.7706, -101.0994) (16.7978, -101.1162) (16.7999, -101.1134) knots 0 0 0 0 1 1 1 1
  spline S2346 degree 3 poles (16.7999, -101.1134) (16.8021, -101.1106) (16.8111, -101.0819) (16.8224, -101.0503) knots 0 0 0 0 1 1 1 1
  spline S2347 degree 3 poles (16.8224, -101.0503) (16.8367, -101.0033) (16.8284, -100.9968) (16.7689, -101.0041) knots 0 0 0 0 1 1 1 1
  spline S2348 degree 3 poles (16.7689, -101.0041) (16.6798, -101.0151) (16.6733, -101.0234) (16.74, -101.0755) knots 0 0 0 0 1 1 1 1
  spline S2349 degree 3 poles (16.382, -101.5166) (16.4071, -101.4959) (16.4418, -101.4514) (16.458, -101.4193) knots 0 0 0 0 1 1 1 1
  spline S2350 degree 3 poles (16.458, -101.4193) (16.4692, -101.3878) (16.4463, -101.4056) (16.405, -101.4585) knots 0 0 0 0 1 1 1 1
  spline S2351 degree 3 poles (16.405, -101.4585) (16.3637, -101.5113) (16.3519, -101.5379) (16.382, -101.5166) knots 0 0 0 0 1 1 1 1
  spline S2352 degree 3 poles (16.5835, -101.3159) (16.6086, -101.2952) (16.6434, -101.2508) (16.6595, -101.2186) knots 0 0 0 0 1 1 1 1
  spline S2353 degree 3 poles (16.6595, -101.2186) (16.6708, -101.1871) (16.6478, -101.205) (16.6066, -101.2578) knots 0 0 0 0 1 1 1 1
  spline S2354 degree 3 poles (16.6066, -101.2578) (16.5653, -101.3106) (16.5535, -101.3372) (16.5835, -101.3159) knots 0 0 0 0 1 1 1 1
  spline S2355 degree 3 poles (11.3084, -108.5835) (11.3246, -108.6544) (11.3296, -108.6538) (11.3282, -108.5811) knots 0 0 0 0 1 1 1 1
  spline S2356 degree 3 poles (11.3282, -108.5811) (11.3268, -108.5084) (11.3154, -108.4771) (11.298, -108.4993) knots 0 0 0 0 1 1 1 1
  spline S2357 degree 3 poles (11.298, -108.4993) (11.2937, -108.5049) (11.2986, -108.5445) (11.3084, -108.5835) knots 0 0 0 0 1 1 1 1
  spline S2358 degree 3 poles (10.8739, -109.1797) (10.8795, -109.1841) (10.9191, -109.1792) (10.9603, -109.1666) knots 0 0 0 0 1 1 1 1
  spline S2359 degree 3 poles (10.9603, -109.1666) (11.029, -109.1531) (11.0284, -109.1482) (10.9556, -109.1496) knots 0 0 0 0 1 1 1 1
  spline S2360 degree 3 poles (10.9556, -109.1496) (10.8829, -109.151) (10.8517, -109.1623) (10.8739, -109.1797) knots 0 0 0 0 1 1 1 1
  spline S2361 degree 3 poles (8.8809, -112.189) (8.8865, -112.1933) (8.9261, -112.1885) (8.9673, -112.1759) knots 0 0 0 0 1 1 1 1
  spline S2362 degree 3 poles (8.9673, -112.1759) (9.036, -112.1624) (9.0354, -112.1575) (8.9627, -112.1589) knots 0 0 0 0 1 1 1 1
  spline S2363 degree 3 poles (8.9627, -112.1589) (8.89, -112.1602) (8.8587, -112.1716) (8.8809, -112.189) knots 0 0 0 0 1 1 1 1
  spline S2364 degree 3 poles (11.2974, -109.2107) (11.3165, -109.2435) (11.3314, -109.2417) (11.342, -109.2052) knots 0 0 0 0 1 1 1 1
  spline S2365 degree 3 poles (11.342, -109.2052) (11.3579, -109.1505) (11.3193, -109.1024) (11.2889, -109.1413) knots 0 0 0 0 1 1 1 1
  spline S2366 degree 3 poles (11.2889, -109.1413) (11.278, -109.1552) (11.2845, -109.1871) (11.2974, -109.2107) knots 0 0 0 0 1 1 1 1
  spline S2367 degree 3 poles (9.2798, -112.326) (9.296, -112.3969) (9.301, -112.3963) (9.2996, -112.3236) knots 0 0 0 0 1 1 1 1
  spline S2368 degree 3 poles (9.2996, -112.3236) (9.2982, -112.2509) (9.2868, -112.2196) (9.2694, -112.2418) knots 0 0 0 0 1 1 1 1
  spline S2369 degree 3 poles (9.2694, -112.2418) (9.2651, -112.2474) (9.27, -112.287) (9.2798, -112.326) knots 0 0 0 0 1 1 1 1
  spline S2370 degree 3 poles (7.3032, -114.896) (7.3088, -114.9003) (7.3484, -114.8954) (7.3896, -114.8829) knots 0 0 0 0 1 1 1 1
  spline S2371 degree 3 poles (7.3896, -114.8829) (7.4583, -114.8694) (7.4577, -114.8644) (7.385, -114.8658) knots 0 0 0 0 1 1 1 1
  spline S2372 degree 3 poles (7.385, -114.8658) (7.3123, -114.8672) (7.281, -114.8786) (7.3032, -114.896) knots 0 0 0 0 1 1 1 1
  spline S2373 degree 3 poles (7.8818, -114.9003) (7.8874, -114.9047) (7.927, -114.8998) (7.9682, -114.8872) knots 0 0 0 0 1 1 1 1
  spline S2374 degree 3 poles (7.9682, -114.8872) (8.0369, -114.8737) (8.0363, -114.8688) (7.9636, -114.8702) knots 0 0 0 0 1 1 1 1
  spline S2375 degree 3 poles (7.9636, -114.8702) (7.8909, -114.8716) (7.8596, -114.883) (7.8818, -114.9003) knots 0 0 0 0 1 1 1 1
  spline S2376 degree 3 poles (8.1352, -114.8969) (8.1875, -114.8929) (8.2343, -114.8847) (8.2408, -114.8764) knots 0 0 0 0 1 1 1 1
  spline S2377 degree 3 poles (8.2408, -114.8764) (8.2473, -114.868) (8.2093, -114.8651) (8.157, -114.8691) knots 0 0 0 0 1 1 1 1
  spline S2378 degree 3 poles (8.157, -114.8691) (8.1047, -114.873) (8.0579, -114.8812) (8.0514, -114.8896) knots 0 0 0 0 1 1 1 1
  spline S2379 degree 3 poles (8.0514, -114.8896) (8.0449, -114.8979) (8.0829, -114.9008) (8.1352, -114.8969) knots 0 0 0 0 1 1 1 1
  spline S2380 degree 3 poles (8.5099, -114.8986) (8.5155, -114.9029) (8.5551, -114.8981) (8.5963, -114.8855) knots 0 0 0 0 1 1 1 1
  spline S2381 degree 3 poles (8.5963, -114.8855) (8.665, -114.872) (8.6644, -114.8671) (8.5917, -114.8685) knots 0 0 0 0 1 1 1 1
  spline S2382 degree 3 poles (8.5917, -114.8685) (8.519, -114.8698) (8.4877, -114.8812) (8.5099, -114.8986) knots 0 0 0 0 1 1 1 1
  spline S2383 degree 3 poles (11.3109, -111.6745) (11.3272, -111.7454) (11.3321, -111.7448) (11.3307, -111.6721) knots 0 0 0 0 1 1 1 1
  spline S2384 degree 3 poles (11.3307, -111.6721) (11.3308, -111.6318) (11.3259, -111.5922) (11.3204, -111.5879) knots 0 0 0 0 1 1 1 1
  spline S2385 degree 3 poles (11.3204, -111.5879) (11.2981, -111.5705) (11.2947, -111.6036) (11.3109, -111.6745) knots 0 0 0 0 1 1 1 1
  spline S2386 degree 3 poles (10.9416, -112.1873) (10.9472, -112.1917) (10.9868, -112.1868) (11.0279, -112.1742) knots 0 0 0 0 1 1 1 1
  spline S2387 degree 3 poles (11.0279, -112.1742) (11.0967, -112.1607) (11.0961, -112.1558) (11.0233, -112.1572) knots 0 0 0 0 1 1 1 1
  spline S2388 degree 3 poles (11.0233, -112.1572) (10.9506, -112.1586) (10.9194, -112.1699) (10.9416, -112.1873) knots 0 0 0 0 1 1 1 1
  spline S2389 degree 3 poles (11.1179, -112.1908) (11.1235, -112.1951) (11.1631, -112.1903) (11.2043, -112.1777) knots 0 0 0 0 1 1 1 1
  spline S2390 degree 3 poles (11.2043, -112.1777) (11.273, -112.1642) (11.2724, -112.1593) (11.1997, -112.1606) knots 0 0 0 0 1 1 1 1
  spline S2391 degree 3 poles (11.1997, -112.1606) (11.127, -112.162) (11.0957, -112.1734) (11.1179, -112.1908) knots 0 0 0 0 1 1 1 1
  spline S2392 degree 3 poles (7.1894, -117.4483) (7.1949, -117.4527) (7.2346, -117.4478) (7.2757, -117.4352) knots 0 0 0 0 1 1 1 1
  spline S2393 degree 3 poles (7.2757, -117.4352) (7.3444, -117.4218) (7.3438, -117.4168) (7.2711, -117.4182) knots 0 0 0 0 1 1 1 1
  spline S2394 degree 3 poles (7.2711, -117.4182) (7.1984, -117.4196) (7.1671, -117.431) (7.1894, -117.4483) knots 0 0 0 0 1 1 1 1
  spline S2395 degree 3 poles (7.4428, -117.4449) (7.4951, -117.441) (7.5418, -117.4327) (7.5483, -117.4244) knots 0 0 0 0 1 1 1 1
  spline S2396 degree 3 poles (7.5483, -117.4244) (7.5549, -117.416) (7.5168, -117.4132) (7.4645, -117.4171) knots 0 0 0 0 1 1 1 1
  spline S2397 degree 3 poles (7.4645, -117.4171) (7.4122, -117.421) (7.3655, -117.4292) (7.359, -117.4376) knots 0 0 0 0 1 1 1 1
  spline S2398 degree 3 poles (7.359, -117.4376) (7.3524, -117.4459) (7.3905, -117.4488) (7.4428, -117.4449) knots 0 0 0 0 1 1 1 1
  spline S2399 degree 3 poles (9.2823, -115.417) (9.2986, -115.4879) (9.3035, -115.4873) (9.3021, -115.4146) knots 0 0 0 0 1 1 1 1
  spline S2400 degree 3 poles (9.3021, -115.4146) (9.3007, -115.3419) (9.2893, -115.3106) (9.272, -115.3328) knots 0 0 0 0 1 1 1 1
  spline S2401 degree 3 poles (9.272, -115.3328) (9.2676, -115.3384) (9.2725, -115.378) (9.2823, -115.417) knots 0 0 0 0 1 1 1 1
  spline S2402 degree 3 poles (7.8175, -117.4466) (7.823, -117.451) (7.8627, -117.4461) (7.9038, -117.4335) knots 0 0 0 0 1 1 1 1
  spline S2403 degree 3 poles (7.9038, -117.4335) (7.9725, -117.42) (7.9719, -117.4151) (7.8992, -117.4165) knots 0 0 0 0 1 1 1 1
  spline S2404 degree 3 poles (7.8992, -117.4165) (7.8265, -117.4179) (7.7952, -117.4292) (7.8175, -117.4466) knots 0 0 0 0 1 1 1 1
  spline S2405 degree 3 poles (8.2197, -117.4475) (8.2253, -117.4518) (8.2649, -117.447) (8.3061, -117.4344) knots 0 0 0 0 1 1 1 1
  spline S2406 degree 3 poles (8.3061, -117.4344) (8.3748, -117.4209) (8.3742, -117.416) (8.3015, -117.4173) knots 0 0 0 0 1 1 1 1
  spline S2407 degree 3 poles (8.3015, -117.4173) (8.2287, -117.4187) (8.1975, -117.4301) (8.2197, -117.4475) knots 0 0 0 0 1 1 1 1
  spline S2408 degree 3 poles (8.6219, -117.4484) (8.6275, -117.4527) (8.6671, -117.4478) (8.7083, -117.4352) knots 0 0 0 0 1 1 1 1
  spline S2409 degree 3 poles (8.7083, -117.4352) (8.777, -117.4218) (8.7764, -117.4168) (8.7037, -117.4182) knots 0 0 0 0 1 1 1 1
  spline S2410 degree 3 poles (8.7037, -117.4182) (8.631, -117.4196) (8.5997, -117.431) (8.6219, -117.4484) knots 0 0 0 0 1 1 1 1
  spline S2411 degree 3 poles (9.2823, -116.8496) (9.2985, -116.9204) (9.3035, -116.9198) (9.3021, -116.8471) knots 0 0 0 0 1 1 1 1
  spline S2412 degree 3 poles (9.3021, -116.8471) (9.3022, -116.8069) (9.2973, -116.7673) (9.2917, -116.7629) knots 0 0 0 0 1 1 1 1
  spline S2413 degree 3 poles (9.2917, -116.7629) (9.2695, -116.7456) (9.266, -116.7787) (9.2823, -116.8496) knots 0 0 0 0 1 1 1 1
  spline S2414 degree 3 poles (9.2814, -117.2518) (9.2976, -117.3227) (9.3026, -117.3221) (9.3012, -117.2493) knots 0 0 0 0 1 1 1 1
  spline S2415 degree 3 poles (9.3012, -117.2493) (9.3013, -117.2091) (9.2964, -117.1695) (9.2909, -117.1652) knots 0 0 0 0 1 1 1 1
  spline S2416 degree 3 poles (9.2909, -117.1652) (9.2686, -117.1478) (9.2652, -117.1809) (9.2814, -117.2518) knots 0 0 0 0 1 1 1 1
  spline S2417 degree 3 poles (9.2667, -117.4597) (9.2806, -117.4705) (9.3054, -117.4675) (9.3162, -117.4536) knots 0 0 0 0 1 1 1 1
  spline S2418 degree 3 poles (9.3162, -117.4536) (9.3293, -117.4369) (9.3241, -117.4149) (9.3102, -117.4041) knots 0 0 0 0 1 1 1 1
  spline S2419 degree 3 poles (9.3102, -117.4041) (9.2935, -117.391) (9.2737, -117.3935) (9.2606, -117.4102) knots 0 0 0 0 1 1 1 1
  spline S2420 degree 3 poles (9.2606, -117.4102) (9.2498, -117.4241) (9.25, -117.4466) (9.2667, -117.4597) knots 0 0 0 0 1 1 1 1
  spline S2421 degree 3 poles (7.5186, -119.7201) (7.5241, -119.7244) (7.5638, -119.7196) (7.6049, -119.707) knots 0 0 0 0 1 1 1 1
  spline S2422 degree 3 poles (7.6049, -119.707) (7.6737, -119.6935) (7.673, -119.6886) (7.6003, -119.69) knots 0 0 0 0 1 1 1 1
  spline S2423 degree 3 poles (7.6003, -119.69) (7.5276, -119.6913) (7.4963, -119.7027) (7.5186, -119.7201) knots 0 0 0 0 1 1 1 1
  spline S2424 degree 3 poles (7.8713, -119.7271) (7.8769, -119.7314) (7.9165, -119.7265) (7.9576, -119.7139) knots 0 0 0 0 1 1 1 1
  spline S2425 degree 3 poles (7.9576, -119.7139) (8.0264, -119.7005) (8.0258, -119.6955) (7.953, -119.6969) knots 0 0 0 0 1 1 1 1
  spline S2426 degree 3 poles (7.953, -119.6969) (7.8803, -119.6983) (7.8491, -119.7097) (7.8713, -119.7271) knots 0 0 0 0 1 1 1 1
  spline S2427 degree 3 poles (8.0972, -119.7245) (8.1027, -119.7288) (8.1423, -119.7239) (8.1835, -119.7113) knots 0 0 0 0 1 1 1 1
  spline S2428 degree 3 poles (8.1835, -119.7113) (8.2522, -119.6979) (8.2516, -119.6929) (8.1789, -119.6943) knots 0 0 0 0 1 1 1 1
  spline S2429 degree 3 poles (8.1789, -119.6943) (8.1062, -119.6957) (8.0749, -119.7071) (8.0972, -119.7245) knots 0 0 0 0 1 1 1 1
  spline S2430 degree 3 poles (8.323, -119.7219) (8.3286, -119.7262) (8.3682, -119.7213) (8.4094, -119.7087) knots 0 0 0 0 1 1 1 1
  spline S2431 degree 3 poles (8.4094, -119.7087) (8.4781, -119.6953) (8.4775, -119.6903) (8.4048, -119.6917) knots 0 0 0 0 1 1 1 1
  spline S2432 degree 3 poles (8.4048, -119.6917) (8.3321, -119.6931) (8.3008, -119.7045) (8.323, -119.7219) knots 0 0 0 0 1 1 1 1
  spline S2433 degree 3 poles (9.2814, -118.6843) (9.2976, -118.7552) (9.3026, -118.7546) (9.3012, -118.6819) knots 0 0 0 0 1 1 1 1
  spline S2434 degree 3 poles (9.3012, -118.6819) (9.3013, -118.6417) (9.2964, -118.6021) (9.2908, -118.5977) knots 0 0 0 0 1 1 1 1
  spline S2435 degree 3 poles (9.2908, -118.5977) (9.2686, -118.5803) (9.2651, -118.6134) (9.2814, -118.6843) knots 0 0 0 0 1 1 1 1
  spline S2436 degree 3 poles (8.7253, -119.7227) (8.7308, -119.7271) (8.7704, -119.7222) (8.8116, -119.7096) knots 0 0 0 0 1 1 1 1
  spline S2437 degree 3 poles (8.8116, -119.7096) (8.8803, -119.6962) (8.8797, -119.6912) (8.807, -119.6926) knots 0 0 0 0 1 1 1 1
  spline S2438 degree 3 poles (8.807, -119.6926) (8.7343, -119.694) (8.703, -119.7054) (8.7253, -119.7227) knots 0 0 0 0 1 1 1 1
  spline S2439 degree 3 poles (8.9511, -119.7201) (8.9567, -119.7245) (8.9963, -119.7196) (9.0375, -119.707) knots 0 0 0 0 1 1 1 1
  spline S2440 degree 3 poles (9.0375, -119.707) (9.1062, -119.6936) (9.1056, -119.6886) (9.0329, -119.69) knots 0 0 0 0 1 1 1 1
  spline S2441 degree 3 poles (9.0329, -119.69) (8.9602, -119.6914) (8.9289, -119.7028) (8.9511, -119.7201) knots 0 0 0 0 1 1 1 1
  spline S2442 degree 3 poles (10.8589, -117.4502) (10.8645, -117.4545) (10.9041, -117.4496) (10.9453, -117.437) knots 0 0 0 0 1 1 1 1
  spline S2443 degree 3 poles (10.9453, -117.437) (11.014, -117.4236) (11.0134, -117.4186) (10.9407, -117.42) knots 0 0 0 0 1 1 1 1
  spline S2444 degree 3 poles (10.9407, -117.42) (10.868, -117.4214) (10.8367, -117.4328) (10.8589, -117.4502) knots 0 0 0 0 1 1 1 1
  spline S2445 degree 3 poles (9.2649, -119.6967) (9.2621, -119.7347) (9.271, -119.7462) (9.2862, -119.7267) knots 0 0 0 0 1 1 1 1
  spline S2446 degree 3 poles (9.2862, -119.7267) (9.2992, -119.7101) (9.3049, -119.6742) (9.2975, -119.655) knots 0 0 0 0 1 1 1 1
  spline S2447 degree 3 poles (9.2975, -119.655) (9.2815, -119.6067) (9.2728, -119.6178) (9.2649, -119.6967) knots 0 0 0 0 1 1 1 1
  spline S2448 degree 3 poles (11.3082, -117.1789) (11.3244, -117.2497) (11.3294, -117.2491) (11.328, -117.1764) knots 0 0 0 0 1 1 1 1
  spline S2449 degree 3 poles (11.328, -117.1764) (11.3266, -117.1037) (11.3152, -117.0724) (11.2978, -117.0947) knots 0 0 0 0 1 1 1 1
  spline S2450 degree 3 poles (11.2978, -117.0947) (11.2935, -117.1002) (11.2984, -117.1398) (11.3082, -117.1789) knots 0 0 0 0 1 1 1 1
  spline S2451 degree 3 poles (9.2787, -119.891) (9.295, -119.9619) (9.2999, -119.9613) (9.2985, -119.8886) knots 0 0 0 0 1 1 1 1
  spline S2452 degree 3 poles (9.2985, -119.8886) (9.2986, -119.8484) (9.2938, -119.8088) (9.2882, -119.8044) knots 0 0 0 0 1 1 1 1
  spline S2453 degree 3 poles (9.2882, -119.8044) (9.266, -119.787) (9.2625, -119.8201) (9.2787, -119.891) knots 0 0 0 0 1 1 1 1
  spline S2454 degree 3 poles (11.3125, -118.0328) (11.3287, -118.1037) (11.3337, -118.1031) (11.3323, -118.0304) knots 0 0 0 0 1 1 1 1
  spline S2455 degree 3 poles (11.3323, -118.0304) (11.3309, -117.9577) (11.3195, -117.9264) (11.3022, -117.9486) knots 0 0 0 0 1 1 1 1
  spline S2456 degree 3 poles (11.3022, -117.9486) (11.2978, -117.9542) (11.3027, -117.9938) (11.3125, -118.0328) knots 0 0 0 0 1 1 1 1
  spline S2457 degree 3 poles (10.4106, -119.7143) (10.418, -119.7335) (10.4434, -119.7355) (10.4691, -119.7197) knots 0 0 0 0 1 1 1 1
  spline S2458 degree 3 poles (10.4691, -119.7197) (10.4998, -119.7034) (10.4979, -119.6885) (10.4614, -119.6779) knots 0 0 0 0 1 1 1 1
  spline S2459 degree 3 poles (10.4614, -119.6779) (10.4039, -119.6599) (10.3925, -119.6688) (10.4106, -119.7143) knots 0 0 0 0 1 1 1 1
  spline S2460 degree 3 poles (11.3107, -118.8373) (11.327, -118.9082) (11.3319, -118.9076) (11.3306, -118.8348) knots 0 0 0 0 1 1 1 1
  spline S2461 degree 3 poles (11.3306, -118.8348) (11.3306, -118.7946) (11.3258, -118.755) (11.3202, -118.7507) knots 0 0 0 0 1 1 1 1